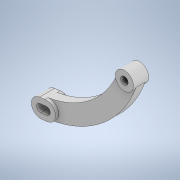
# Autodesk Inventor part: Part5
Saved by Autodesk Inventor 2020 (Build 240168000, 168)
## iProperties
Created: 2019-08-16
Part Number: Part5
Material: Generic
Document SubType Name: Modeling
Designer: Horváth Patrik
Density: 1 g/cm^3
Appearance: Default
Author: Horváth Patrik
Autodesk Inventor part; units mm, degrees
ref_plane "YZ Plane" through (0, 0, 0) normal (1, 0, 0) x (0, 1, 0)
ref_plane "XZ Plane" through (0, 0, 0) normal (0, 1, 0) x (-1, 0, 0)
ref_plane "XY Plane" through (0, 0, 0) normal (0, 0, 1) x (1, 0, 0)
sketch "Sketch1" plane through (0, 0, 0) normal (0, 0, 1) x (1, 0, 0)
  circle A0 centre (5.5, 0) radius 1.4795 projected
  circle A1 centre (32.1927, 21.5482) radius 1.25 projected
  circle A2 centre (5.5, 0) radius 3
  circle A3 centre (32.1927, 21.5482) radius 3
  point P0 (0, 0)
  dimension "d0" = 6
  constraints: 2 centre point, 2 coincident, 1 equal radius
  measures "d0" diameter of A2
extrude "Extrusion1" add sketch "Sketch1" along normal blind 1
sketch "Sketch2" plane through (5.5, 0, 1) normal (0, 0, 1) x (1, 0, 0)
  circle A0 centre (0, 0) radius 3 projected
  circle A1 centre (0, 0) radius 1.4795 projected
  circle A2 centre (26.6927, 21.5482) radius 3 projected
  circle A3 centre (26.6927, 21.5482) radius 1.25 projected
  circle A4 centre (26.6927, 21.5482) radius 1.25 projected
  arc A5 (0, 0) -> (26.6927, 21.5482) centre (-4.3622, 32.7104) ccw construction
  arc A6 (0.3966, -2.9737) -> (29.5159, 20.5335) centre (-4.3622, 32.7104) ccw
  arc A7 (-0.3966, 2.9737) -> (23.8695, 22.563) centre (-4.3622, 32.7104) ccw
  arc A8 (-0.3966, 2.9737) -> (0.3966, -2.9737) centre (0, 0) ccw
  arc A9 (29.5159, 20.5335) -> (23.8695, 22.563) centre (26.6927, 21.5482) ccw
  circle A10 centre (19.7, 21.8678) radius 2.5 projected
  circle A11 centre (0, 0) radius 3 projected
  point P0 (-5.5, 0)
  point P1 (23.8695, 22.563)
  point P2 (-0.3966, 2.9737)
  point P3 (0.3966, -2.9737)
  point P4 (29.5159, 20.5335)
  dimension "d3" = 30
  constraints: 10 point on circle, 5 centre point, 4 tangent, 1 concentric
  measures "d3" radius of A7
extrude "Extrusion2" add sketch "Sketch2" along normal blind 3 contours A0 | A0 A7 A2 A6 | A2
sketch "Sketch3" plane through (5.5, 0, 1) normal (0, 0, -1) x (-1, 0, 0)
  arc A0 (-29.5159, 20.5335) -> (-23.8695, 22.563) centre (-26.6927, 21.5482) ccw construction
  arc A1 (-29.5159, 20.5335) -> (-0.3966, -2.9737) centre (4.3622, 32.7104) ccw construction
  arc A2 (0.3966, 2.9737) -> (-0.3966, -2.9737) centre (0, 0) ccw construction
  arc A3 (-23.8695, 22.563) -> (0.3966, 2.9737) centre (4.3622, 32.7104) ccw construction
  circle A4 centre (0, 0) radius 3 construction
  circle A5 centre (0, 0) radius 1.4795 construction
  arc A6 (-1, 0.149) -> (1, -0.1179) centre (4.3622, 32.7104) ccw construction
  arc A7 (-1.4875, -2.8111) -> (0.6943, -3.1022) centre (4.3622, 32.7104) ccw
  arc A8 (-0.5125, 3.1091) -> (1.3057, 2.8665) centre (4.3622, 32.7104) ccw
  arc A9 (-0.5125, 3.1091) -> (-1.4875, -2.8111) centre (-1, 0.149) ccw
  arc A10 (0.6943, -3.1022) -> (1.3057, 2.8665) centre (1, -0.1179) ccw
  point P0 (5.5, 0)
  dimension "d6" = 1
  dimension "d7" = 1
  constraints: 10 point on circle, 6 tangent, 5 centre point, 1 concentric
  measures "d6" horizontal distance of A6.end A2.centre
  measures "d7" horizontal distance of A6.start A2.centre
extrude "Extrusion3" add sketch "Sketch3" along normal blind 1 and the other way blind 4
sketch "Sketch4" plane through (5.5, 0, 4) normal (0, 0, 1) x (1, 0, 0)
  arc A0 (29.5159, 20.5335) -> (23.8695, 22.563) centre (26.6927, 21.5482) ccw projected
  circle A1 centre (26.6927, 21.5482) radius 1.25 projected
  circle A2 centre (26.6927, 21.5482) radius 3 projected
  circle A3 centre (26.6927, 21.5482) radius 3
  point P0 (-5.5, 0)
  constraints: 1 centre point, 1 coincident, 1 concentric
extrude "Extrusion4" add sketch "Sketch4" along normal blind 1
sketch "Sketch5" plane through (0, 0, 0) normal (0, 0, -1) x (-1, 0, 0)
  arc A0 (-6.9875, -2.8111) -> (-4.8057, -3.1022) centre (-1.1378, 32.7104) ccw projected
  arc A1 (-4.8057, -3.1022) -> (-4.1943, 2.8665) centre (-4.5, -0.1179) ccw projected
  arc A2 (-6.0125, 3.1091) -> (-4.1943, 2.8665) centre (-1.1378, 32.7104) ccw projected
  arc A3 (-6.0125, 3.1091) -> (-6.9875, -2.8111) centre (-6.5, 0.149) ccw projected
  arc A4 (-6.5, 0.149) -> (-4.5, -0.1179) centre (-1.1378, 32.7104) ccw construction
  arc A5 (-6.7031, -1.0844) -> (-4.6274, -1.3614) centre (-1.1378, 32.7104) ccw
  arc A6 (-6.2969, 1.3824) -> (-4.3726, 1.1256) centre (-1.1378, 32.7104) ccw
  arc A7 (-6.2969, 1.3824) -> (-6.7031, -1.0844) centre (-6.5, 0.149) ccw
  arc A8 (-4.6274, -1.3614) -> (-4.3726, 1.1256) centre (-4.5, -0.1179) ccw
  arc A9 (-6.9875, -2.8111) -> (-4.8057, -3.1022) centre (-1.1378, 32.7104) ccw projected
  point P0 (0, 0)
  dimension "d14" = 2.5
  constraints: 10 point on circle, 5 centre point, 4 tangent, 1 coincident, 1 concentric
  measures "d14" radial gap between concentric circles of A5 A6
extrude "Extrusion5" cut sketch "Sketch5" against normal blind 5 contours A7 A6 A8 A5
equation "\"d7\" = d6"
body "Solid1"
